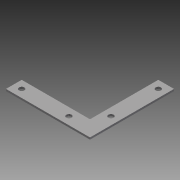
# Autodesk Inventor part: wood gusset
Saved by Autodesk Inventor 2015 SP1 (Build 190203100, 203)
## iProperties
Created: 2015-01-31
Part Number: wood gusset
Material: Generic
Document SubType Name: Modeling
Designer: Admin
Density: 1 g/cm^3
Appearance: Default
Author: Admin
Autodesk Inventor part; units mm, degrees
ref_plane "YZ Plane" through (0, 0, 0) normal (1, 0, 0) x (0, 1, 0)
ref_plane "XZ Plane" through (0, 0, 0) normal (0, 1, 0) x (-1, 0, 0)
ref_plane "XY Plane" through (0, 0, 0) normal (0, 0, 1) x (1, 0, 0)
sketch "Sketch1" plane through (0, 0, 0) normal (0, 1, 0) x (-1, 0, 0)
  line L0 (0, 0) -> (101.6, 0)
  line L1 (101.6, 0) -> (101.6, -19.05)
  line L2 (101.6, -19.05) -> (0, -19.05)
  line L3 (0, -19.05) -> (0, 0)
  line L4 (0, 0) -> (19.05, 0)
  line L5 (19.05, 0) -> (19.05, -101.6)
  line L6 (19.05, -101.6) -> (0, -101.6)
  line L7 (0, -101.6) -> (0, 0)
  dimension "d0" = 101.6
  dimension "d1" = 19.05
  dimension "d2" = 19.05
  dimension "d3" = 101.6
  constraints: 16 end point, 4 parallel, 2 horizontal, 2 perpendicular
  measures "d0" distance of L1.end L2.end
  measures "d1" distance of L0.end L1.end
  measures "d2" distance of L5.end L6.end
  measures "d3" distance of L4.end L5.end
extrude "Extrusion1" add sketch "Sketch1" along normal blind 2.286
sketch "Sketch2" plane through (0, 2.286, 0) normal (0, 1, 0) x (1, 0, 0)
  line L0 (0, 0) -> (0, 101.6) projected
  line L1 (-101.6, 0) -> (0, 0) projected
  point P0 (-34.925, 9.525)
  point P1 (-92.075, 9.525)
  point P2 (-9.525, 34.925)
  point P3 (-9.525, 92.075)
  dimension "d8" = 9.525
  dimension "d11" = 9.525
  dimension "d13" = 9.525
  dimension "d14" = 9.525
  dimension "d23" = 34.925
  dimension "d24" = 92.075
  dimension "d25" = 34.925
  dimension "d26" = 92.075
  measures "d8" distance from line of L1 point (-34.925, 9.525)
  measures "d11" distance from line of L1 point (-92.075, 9.525)
  measures "d13" distance from line of L0 point (-9.525, 34.925)
  measures "d14" distance from line of L0 point (-9.525, 92.075)
  measures "d23" distance from line of point (-9.525, 34.925) L1
  measures "d24" distance from line of point (-9.525, 92.075) L1
  measures "d25" distance from line of L0 point (-34.925, 9.525)
  measures "d26" distance from line of point (-92.075, 9.525) L0
hole "Hole1" at (-34.925, 2.286, -9.525) at (-92.075, 2.286, -9.525) at (-9.525, 2.286, -34.925) at (-9.525, 2.286, -92.075) direction (0, -1, 0) diameter 6.35 end through all
body "Solid1"
